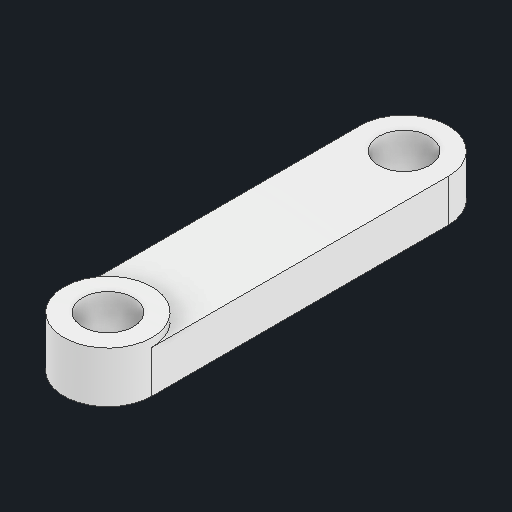
# Autodesk Inventor part: wiper_linkage_motor_connect
Saved by Autodesk Inventor 2026.2 (Build 302298000, 298)
## iProperties
Created: 2026-03-09
Part Number: wiper_linkage_motor_connect
Material: ABS Plastic
Document SubType Name: Modeling
Designer: Tathagata Sikdar
Density: 1.06 g/cm^3
Appearance: Smooth - White
Author: Tathagata Sikdar
Autodesk Inventor part; units mm, degrees
ref_plane "YZ Plane" through (0, 0, 0) normal (1, 0, 0) x (0, 1, 0)
ref_plane "XZ Plane" through (0, 0, 0) normal (0, 1, 0) x (-1, 0, 0)
ref_plane "XY Plane" through (0, 0, 0) normal (0, 0, 1) x (1, 0, 0)
sketch "Sketch1" plane through (0, 0, 0) normal (0, 1, 0) x (-1, 0, 0)
  line L0 (0, 0) -> (0, -45) construction
  line L1 (-5, -5) -> (-5, -40) construction
  line L2 (5, -40) -> (5, -5) construction
  arc A0 (5, -5) -> (-5, -5) centre (0, -5) ccw construction
  arc A1 (-5, -40) -> (5, -40) centre (0, -40) ccw construction
  line L3 (-5.2, -40) -> (-5.2, -5)
  arc A2 (5.2, -5) -> (-5.2, -5) centre (0, -5) ccw
  line L4 (5.2, -5) -> (5.2, -40)
  arc A3 (-5.2, -40) -> (5.2, -40) centre (0, -40) ccw
  circle A4 centre (0, -5) radius 3
  circle A5 centre (0, -40) radius 3
  circle A6 centre (0, -5) radius 5.2
  point P0 (0, -22.5)
  dimension "d0" = 45
  dimension "d1" = 10
  dimension "d2" = 0.2
  dimension "d3" = 6
  dimension "d4" = 6
  constraints: 12 end point, 10 point on circle, 7 centre point, 5 tangent, 3 coincident, 2 parallel, 2 point on line, 1 midpoint, 1 vertical, 3 other
  measures "d0" distance of L0.start L0.end
  measures "d1" diameter of A1
  measures "d2" distance between parallel lines of L1 L3
  measures "d3" diameter of A4
  measures "d4" diameter of A5
extrude "Extrusion1" add sketch "Sketch1" along normal blind 5 contours L3 A6 L4 A3
extrude "Extrusion2" add sketch "Sketch1" along normal blind 6 contours A2 A6
body "Solid1"
